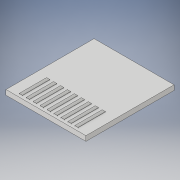
# Autodesk Inventor part: PCB
Saved by Autodesk Inventor 2019 (Build 230136000, 136)
## iProperties
Created: 2019-02-19
Part Number: PCB
Material: 일반
Document SubType Name: Modeling
Designer: Jeong Ji Hoon
Density: 1 g/cm^3
Appearance: 기본값
Author: Jeong Ji Hoon
Autodesk Inventor part; units mm, degrees
ref_plane "YZ Plane" through (0, 0, 0) normal (1, 0, 0) x (0, 1, 0)
ref_plane "XZ Plane" through (0, 0, 0) normal (0, 1, 0) x (-1, 0, 0)
ref_plane "XY Plane" through (0, 0, 0) normal (0, 0, 1) x (1, 0, 0)
sketch "스케치1" plane through (0, 0, 0) normal (0, 1, 0) x (-1, 0, 0)
  line L0 (0, 0) -> (14.6, 0)
  line L1 (14.6, 0) -> (14.6, -16.1)
  line L2 (14.6, -16.1) -> (0, -16.1)
  line L3 (0, -16.1) -> (0, 0)
  dimension "d0" = 14.6
  dimension "d1" = 16.1
  constraints: 8 end point, 2 parallel, 1 horizontal, 1 perpendicular
  measures "d0" distance of L1.end L2.end
  measures "d1" distance of L0.end L1.end
extrude "돌출1" add sketch "스케치1" along normal blind 0.9
sketch "스케치2" plane through (0, 0.9, 0) normal (0, 1, 0) x (1, 0, 0)
  line L0 (-12.68, 0.5) -> (-12.08, 0.5)
  line L1 (-12.08, 0.5) -> (-12.08, 5.5)
  line L2 (-12.08, 5.5) -> (-12.68, 5.5)
  line L3 (-12.68, 5.5) -> (-12.68, 0.5)
  line L4 (-14.6, 0) -> (0, 0) projected
  line L5 (-14.6, 16.1) -> (-14.6, 0) projected
  line L6 (-11.41, 0.5) -> (-10.81, 0.5)
  line L7 (-10.81, 0.5) -> (-10.81, 5.5)
  line L8 (-10.81, 5.5) -> (-11.41, 5.5)
  line L9 (-11.41, 5.5) -> (-11.41, 0.5)
  line L10 (-10.14, 0.5) -> (-9.54, 0.5)
  line L11 (-9.54, 0.5) -> (-9.54, 5.5)
  line L12 (-9.54, 5.5) -> (-10.14, 5.5)
  line L13 (-10.14, 5.5) -> (-10.14, 0.5)
  line L14 (-8.87, 0.5) -> (-8.27, 0.5)
  line L15 (-8.27, 0.5) -> (-8.27, 5.5)
  line L16 (-8.27, 5.5) -> (-8.87, 5.5)
  line L17 (-8.87, 5.5) -> (-8.87, 0.5)
  line L18 (-7.6, 0.5) -> (-7, 0.5)
  line L19 (-7, 0.5) -> (-7, 5.5)
  line L20 (-7, 5.5) -> (-7.6, 5.5)
  line L21 (-7.6, 5.5) -> (-7.6, 0.5)
  line L22 (-6.33, 0.5) -> (-5.73, 0.5)
  line L23 (-5.73, 0.5) -> (-5.73, 5.5)
  line L24 (-5.73, 5.5) -> (-6.33, 5.5)
  line L25 (-6.33, 5.5) -> (-6.33, 0.5)
  line L26 (-5.06, 0.5) -> (-4.46, 0.5)
  line L27 (-4.46, 0.5) -> (-4.46, 5.5)
  line L28 (-4.46, 5.5) -> (-5.06, 5.5)
  line L29 (-5.06, 5.5) -> (-5.06, 0.5)
  line L30 (-3.79, 0.5) -> (-3.19, 0.5)
  line L31 (-3.19, 0.5) -> (-3.19, 5.5)
  line L32 (-3.19, 5.5) -> (-3.79, 5.5)
  line L33 (-3.79, 5.5) -> (-3.79, 0.5)
  line L34 (-2.52, 0.5) -> (-1.92, 0.5)
  line L35 (-1.92, 0.5) -> (-1.92, 5.5)
  line L36 (-1.92, 5.5) -> (-2.52, 5.5)
  line L37 (-2.52, 5.5) -> (-2.52, 0.5)
  line L38 (0, 0) -> (0, 16.1) projected
  dimension "d4" = 0.6
  dimension "d5" = 5
  dimension "d6" = 0.5
  dimension "d7" = 1.92
  dimension "d10" = 1.27
  dimension "d15" = 1.92
  constraints: 72 end point, 2 horizontal, 2 parallel, 1 perpendicular, 64 other
  measures "d4" distance of L2.end L1.end
  measures "d5" distance of L1.end L0.end
  measures "d6" distance between parallel lines of L4 L0
  measures "d7" distance between parallel lines of L5 L3
  measures "d10" distance of L0.start L6.start
  measures "d15" distance between parallel lines of L35 L38
extrude "돌출2" add sketch "스케치2" along normal blind 0.1 and the other way blind 1 separate body
